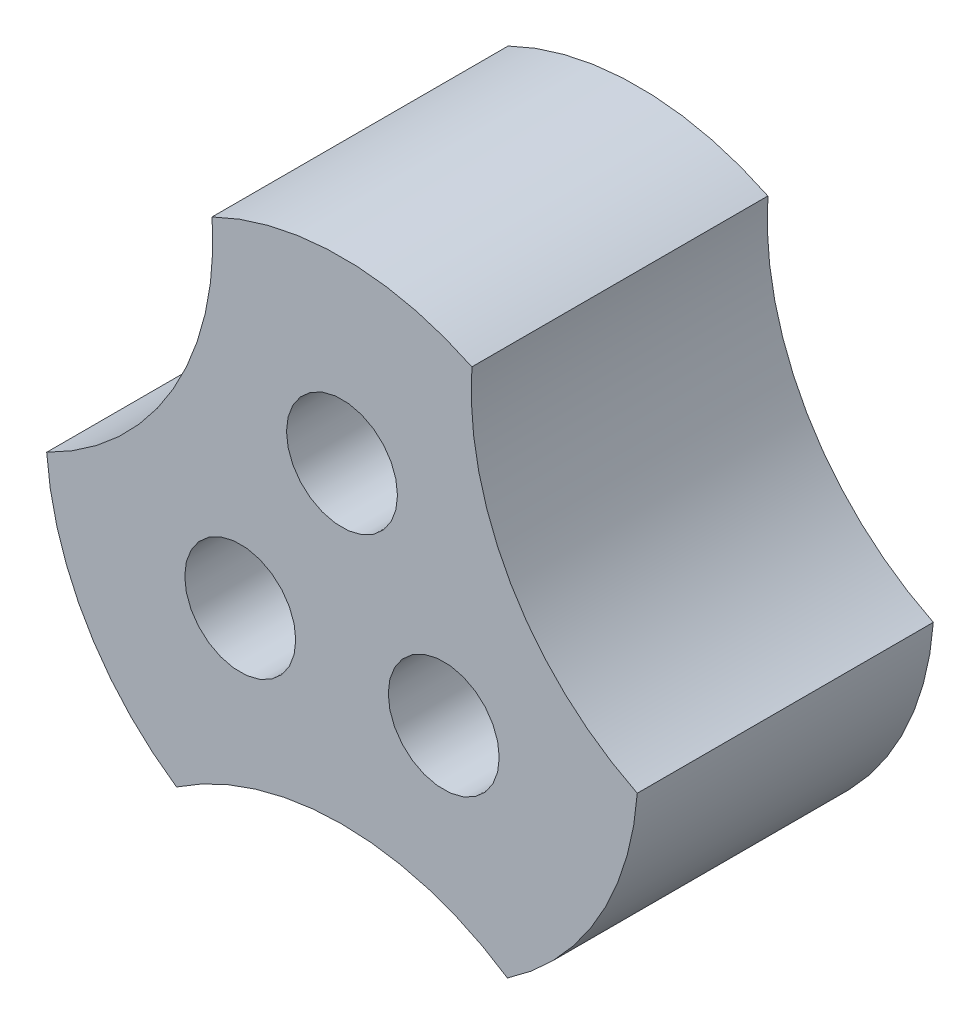
# Autodesk Inventor part: Part3
Saved by Autodesk Inventor 2020 (Build 240168000, 168)
## iProperties
Created: 2020-01-24
Part Number: Part3
Material: 一般
Document SubType Name: Modeling
Designer: tanjihayato
Density: 1 g/cm^3
Appearance: 既定
Author: tanjihayato
Autodesk Inventor part; units mm, degrees
ref_plane "YZ Plane" through (0, 0, 0) normal (1, 0, 0) x (0, 1, 0)
ref_plane "XZ Plane" through (0, 0, 0) normal (0, 1, 0) x (-1, 0, 0)
ref_plane "XY Plane" through (0, 0, 0) normal (0, 0, 1) x (1, 0, 0)
sketch "スケッチ1" plane through (0, 0, 0) normal (0, 0, 1) x (1, 0, 0)
  circle A0 centre (0, 0) radius 8
  line L0 (0, 3.1754) -> (2.75, -1.5877) construction
  line L1 (2.75, -1.5877) -> (-2.75, -1.5877) construction
  line L2 (-2.75, -1.5877) -> (0, 3.1754) construction
  circle A1 centre (0, 3.1754) radius 1.5
  circle A2 centre (2.75, -1.5877) radius 1.5
  circle A3 centre (-2.75, -1.5877) radius 1.5
  circle A4 centre (0, 3.1754) radius 4
  circle A5 centre (2.75, -1.5877) radius 4
  circle A6 centre (-2.75, -1.5877) radius 4
  arc A7 (-7.9807, -0.5547) -> (-3.51, 7.1889) centre (-11.4907, 6.6342) ccw
  arc A8 (3.51, 7.1889) -> (7.9807, -0.5547) centre (11.4907, 6.6342) ccw
  arc A9 (4.4708, -6.6342) -> (-4.4708, -6.6342) centre (0, -13.2684) ccw
  dimension "d0" = 16
  dimension "d1" = 5.5
  dimension "d2" = 3
  dimension "d3" = 3
  dimension "d4" = 3
  dimension "d5" = 2.5
  dimension "d6" = 2.5
  dimension "d7" = 2.5
  dimension "d8" = 8
  dimension "d9" = 8
  dimension "d10" = 8
  constraints: 12 point on circle, 10 centre point, 6 end point, 6 tangent, 5 coincident, 1 horizontal, 7 other
  measures "d0" diameter of A0
  measures "d1" distance of L0.end L1.end
  measures "d2" diameter of A1
  measures "d3" diameter of A2
  measures "d4" diameter of A3
  measures "d5" radial gap between concentric circles of A1 A4
  measures "d6" radial gap between concentric circles of A2 A5
  measures "d7" radial gap between concentric circles of A3 A6
  measures "d8" radius of A8
  measures "d9" radius of A7
  measures "d10" radius of A9
extrude "押し出し1" add sketch "スケッチ1" along normal blind 8 contours A8 A4 A7 A0 | A0 A9 A5 A8 | A8 A5 A4 | A4 A5 A1 A6 | A5 A6 A2 A4 | A7 A6 A9 A0 | A4 A6 A7 | A9 A6 A5 | A4 A6 A5 | A6 A4 A3 A5 | A6 A5 A4 | A5 A4 A6 | A2 A6 A4 | A5 A6 A1 | A4 A5 A3 | A4 A5 A6
